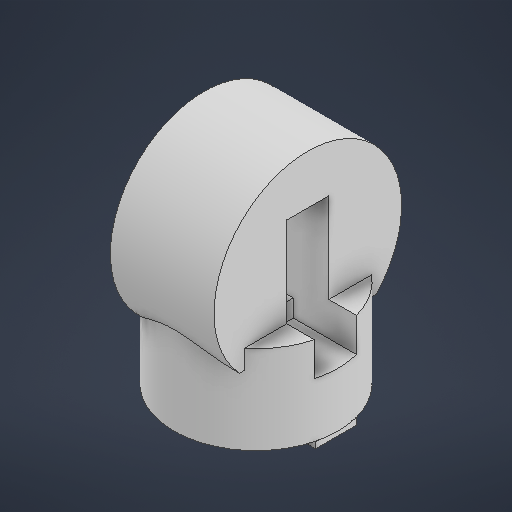
# Autodesk Inventor part: bottomPart
Saved by Autodesk Inventor 2026.2 (Build 302298000, 298)
## iProperties
Created: 2026-04-05
Part Number: bottomPart
Material: Generic
Document SubType Name: Modeling
Designer: Brian Wang
Density: 1 g/cm^3
Appearance: Default
Author: Brian Wang
Autodesk Inventor part; units mm, degrees
ref_plane "YZ Plane" through (0, 0, 0) normal (1, 0, 0) x (0, 1, 0)
ref_plane "XZ Plane" through (0, 0, 0) normal (0, 1, 0) x (-1, 0, 0)
ref_plane "XY Plane" through (0, 0, 0) normal (0, 0, 1) x (1, 0, 0)
sketch "Sketch1" plane through (0, 0, 0) normal (0, 1, 0) x (-1, 0, 0)
  line L0 (39, 10) -> (10, 10)
  line L1 (10, 10) -> (10, 30)
  line L2 (10, 30) -> (-10, 30)
  line L3 (-10, 30) -> (-10, 10)
  line L4 (-10, 10) -> (-39, 10)
  line L5 (-39, 10) -> (-39, -10)
  line L6 (-39, -10) -> (-10, -10)
  line L7 (-10, -10) -> (-10, -30)
  line L8 (-10, -30) -> (10, -30)
  line L9 (10, -30) -> (10, -10)
  line L10 (39, -10) -> (10, -10)
  line L11 (39, -10) -> (39, 10)
  circle A0 centre (25, 5) radius 1.375
  circle A1 centre (-25, 5) radius 1.375
  circle A2 centre (25, -5) radius 1.375
  circle A3 centre (-25, -5) radius 1.375
  point P0 (0, 0)
  dimension "d0" = 29
  dimension "d1" = 20
  dimension "d2" = 90
  dimension "d3" = 20
  dimension "d4" = 90
  dimension "d5" = 29
  dimension "d6" = 20
  dimension "d7" = 90
  dimension "d8" = 20
  dimension "d11" = 2.75
  dimension "d12" = 2.75
  dimension "d13" = 50
  dimension "d14" = 78
  dimension "d15" = 14
  dimension "d16" = 5
  dimension "d20" = 14
  dimension "d21" = 5
  dimension "d22" = 10
  dimension "d23" = 14
  dimension "d24" = 5
  dimension "d25" = 10
  dimension "d26" = 5
  constraints: 24 end point, 8 perpendicular, 8 point on line, 4 centre point, 1 horizontal
  measures "d0" distance of L0.start L0.end
  measures "d1" distance of L0.end L1.end
  measures "d2" angle of L0 L1
  measures "d3" distance of L1.end L2.end
  measures "d4" angle of L2 L1
  measures "d5" distance of L3.end L4.end
  measures "d6" distance of L4.end L5.end
  measures "d7" angle of L5 L4
  measures "d8" distance of L6.end L7.end
  measures "d11" diameter of A0
  measures "d12" diameter of A1
  measures "d13" distance of A1.centre A0.centre
  measures "d14" distance between parallel lines of L11 L5
  measures "d15" distance from line of L11 A0.centre
  measures "d16" distance from line of L0 A0.centre
  measures "d20" distance from line of L11 A2.centre
  measures "d21" distance from line of L10 A2.centre
  measures "d22" distance of A0.centre A2.centre
  measures "d23" distance from line of L5 A3.centre
  measures "d24" distance from line of L6 A3.centre
  measures "d25" distance of A3.centre A1.centre
  measures "d26" distance from line of L4 A1.centre
extrude "Extrusion1" add sketch "Sketch1" along normal blind 3
sketch "Sketch2" plane through (0, 3, 0) normal (0, 1, 0) x (1, 0, 0)
  circle A0 centre (0, 0) radius 40
  dimension "d27" = 80
  constraints: 1 centre point, 1 coincident
  measures "d27" diameter of A0
extrude "Extrusion2" add sketch "Sketch2" along normal blind 3
sketch "Sketch3" plane through (0, 6, 0) normal (0, 1, 0) x (1, 0, 0)
  circle A0 centre (0, 0) radius 40
  circle A1 centre (0, 0) radius 36.5
  dimension "d31" = 73
  constraints: 2 centre point, 2 coincident
  measures "d31" diameter of A1
extrude "Extrusion3" add sketch "Sketch3" along normal blind 40 contours A0 | A1
sketch "Sketch4" plane through (0, 46, 0) normal (0, 1, 0) x (1, 0, 0)
  line L0 (-19.25, 10.25) -> (19.25, 10.25)
  line L1 (19.25, 10.25) -> (19.25, -10.25)
  line L2 (19.25, -10.25) -> (-19.25, -10.25)
  line L3 (-19.25, -10.25) -> (-19.25, 10.25)
  point P0 (0, 0)
  dimension "d34" = 38.5
  dimension "d35" = 20.5
  dimension "d36" = 19.25
  dimension "d37" = 10.25
  constraints: 8 end point, 2 parallel, 1 horizontal, 1 perpendicular
  measures "d34" distance of L1.end L2.end
  measures "d35" distance of L0.end L1.end
  measures "d36" distance from line of L3 point (0, 0)
  measures "d37" distance from line of L0 point (0, 0)
extrude "Extrusion4" cut sketch "Sketch4" against normal blind 8
sketch "Sketch5" plane through (0, 38, 0) normal (0, 1, 0) x (1, 0, 0)
  line L0 (-19.25, 10.25) -> (19.25, 10.25) projected
  line L1 (19.25, -10.25) -> (-19.25, -10.25) projected
  line L2 (10.8, 10.25) -> (7.9, 10.25)
  line L3 (7.9, 10.25) -> (7.9, -10.25)
  line L4 (7.9, -10.25) -> (10.8, -10.25)
  line L5 (10.8, -10.25) -> (10.8, 10.25)
  line L6 (19.25, 10.25) -> (19.25, -10.25) projected
  line L7 (6.4, -10.25) -> (3.84, -10.25)
  line L8 (3.84, 10.25) -> (6.4, 10.25)
  point P0 (0, 0)
  dimension "d40" = 2.9
  dimension "d41" = 8.45
  constraints: 12 end point, 4 point on line, 3 parallel, 2 horizontal, 1 perpendicular
  measures "d40" distance of L4.end L3.end
  measures "d41" distance between parallel lines of L6 L5
extrude "Extrusion5" cut sketch "Sketch5" against normal blind 8.5 contours L0 L5 L1 L3
sketch "Sketch6" plane through (7.9, 38, 10.25) normal (1, 0, 0) x (0, 0, -1)
  line L0 (0, 0) -> (0, -8.5) projected
  line L1 (0, 0) -> (20.5, 0) projected
  line L2 (0, -8.5) -> (20.5, -8.5)
  line L3 (20.5, -8.5) -> (20.5, 0)
  line L4 (20.5, 0) -> (0, 0)
  line L5 (0, 0) -> (0, -8.5)
  point P0 (10.25, -38)
  constraints: 8 end point, 2 parallel, 1 horizontal, 1 perpendicular
extrude "Extrusion6" cut sketch "Sketch6" along normal blind 49
sketch "Sketch7" plane through (7.9, 38, 10.25) normal (1, 0, 0) x (0, 0, -1)
  circle A0 centre (5.25, -4.25) radius 1.35
  circle A1 centre (15.25, -4.25) radius 1.35
  line L0 (20.5, 0) -> (0, 0) projected
  line L1 (0, -8.5) -> (0, 0) projected
  point P0 (10.25, -38)
  dimension "d48" = 2.7
  dimension "d49" = 2.7
  dimension "d50" = 10
  dimension "d51" = 4.25
  dimension "d52" = 4.25
  dimension "d53" = 5.25
  constraints: 2 centre point
  measures "d48" diameter of A0
  measures "d49" diameter of A1
  measures "d50" distance of A0.centre A1.centre
  measures "d51" distance from line of L0 A0.centre
  measures "d52" distance from line of L0 A1.centre
  measures "d53" distance from line of L1 A0.centre
extrude "Extrusion7" cut sketch "Sketch7" against normal blind 7
sketch "Sketch8" plane through (0, 0, 0) normal (1, 0, 0) x (0, 1, 0)
  circle A0 centre (68, 0) radius 45.7097
  line L0 (29.5, 10.25) -> (29.5, -10.25) projected
  line L1 (29.5, -10.25) -> (77.6, -10.25)
  line L2 (77.6, -10.25) -> (77.6, 10.25)
  line L3 (77.6, 10.25) -> (29.5, 10.25)
  line L4 (29.5, 10.25) -> (29.5, -10.25)
  circle A1 centre (68, 0) radius 2.5
  point P0 (0, 0)
  dimension "d56" = 48.1
  dimension "d74" = 5
  constraints: 8 end point, 2 centre point, 2 parallel, 1 coincident, 1 horizontal, 1 perpendicular
  measures "d56" distance of L3.end L2.end
  measures "d74" diameter of A1
extrude "Extrusion8" add sketch "Sketch8" along normal mid plane 44.5 contours A0
sketch "Sketch9" plane through (0, 29.5, 0) normal (0, 1, 0) x (1, 0, 0)
  line L0 (22.25, -10.25) -> (22.25, 10.25) projected
  line L1 (7.9, -10.25) -> (7.9, 10.25) projected
  line L2 (22.25, 10.25) -> (7.9, 10.25)
  line L3 (7.9, 10.25) -> (7.9, -10.25)
  line L4 (7.9, -10.25) -> (22.25, -10.25)
  line L5 (22.25, -10.25) -> (22.25, 10.25)
  point P0 (0, 0)
  point P1 (22.25, -10.25)
  constraints: 8 end point, 2 parallel, 1 horizontal, 1 perpendicular
extrude "Extrusion9" cut sketch "Sketch9" along normal blind 56.1
sketch "Sketch10" plane through (0, 29.5, 0) normal (0, 1, 0) x (1, 0, 0)
  line L0 (22.25, 10.25) -> (22.25, -10.25) projected
  line L1 (22.25, -10.25) -> (93.4732, -10.25)
  line L2 (93.4732, -10.25) -> (93.4732, 10.25)
  line L3 (93.4732, 10.25) -> (22.25, 10.25)
  line L4 (22.25, 10.25) -> (22.25, -10.25)
  point P0 (0, 0)
  point P1 (22.25, 10.25)
  constraints: 8 end point, 2 parallel, 1 horizontal, 1 perpendicular
extrude "Extrusion10" cut sketch "Sketch10" along normal blind 32.85
sketch "Sketch11" plane through (7.9, 77.6, -10.25) normal (1, 0, 0) x (0, 0, -1)
  circle A0 centre (-15.25, -43.85) radius 1.35 projected
  circle A1 centre (-15.25, -43.85) radius 1.35
  circle A2 centre (-5.25, -43.85) radius 1.35 projected
  circle A3 centre (-5.25, -43.85) radius 1.35
  circle A4 centre (-15.25, 6.15) radius 1.35
  circle A5 centre (-5.25, 6.15) radius 1.35
  point P0 (-10.25, -77.6)
  dimension "d63" = 2.7
  dimension "d64" = 50
  dimension "d65" = 50
  constraints: 4 centre point, 2 coincident
  measures "d63" diameter of A4
  measures "d64" distance of A1.centre A4.centre
  measures "d65" distance of A3.centre A5.centre
sketch "Sketch12" plane through (22.25, 0, 0) normal (1, 0, 0) x (0, 0, -1)
  line L0 (-10.25, 85.6) -> (10.25, 85.6) projected
  line L1 (-10.25, 85.6) -> (10.25, 85.6)
  line L2 (10.25, 85.6) -> (10.25, 89.7782)
  line L3 (10.25, 89.7782) -> (-10.25, 89.7782)
  line L4 (-10.25, 89.7782) -> (-10.25, 85.6)
  point P0 (0, 0)
  constraints: 8 end point, 2 parallel, 1 horizontal, 1 perpendicular
sketch "Sketch13" plane through (7.9, 77.6, -10.25) normal (1, 0, 0) x (0, 0, -1)
  line L0 (0, 0) -> (-20.5, 0) projected
  line L1 (-20.5, -31.6) -> (-20.5, 8) projected
  line L2 (0, 0) -> (-20.5, 0)
  line L3 (-20.5, 0) -> (-20.5, 2.8423)
  line L4 (-20.5, 2.8423) -> (0, 2.8423)
  line L5 (0, 2.8423) -> (0, 0)
  point P0 (-10.25, -77.6)
  constraints: 8 end point, 2 parallel, 1 horizontal, 1 perpendicular, 1 point on line
extrude "Extrusion11" cut sketch "Sketch13" against normal blind 65.65
extrude "Extrusion12" cut sketch "Sketch12" against normal up to surface (14.35 mm away)
extrude "Extrusion13" cut sketch "Sketch11" against normal blind 7 contours A4 | A5
sketch "Sketch14" plane through (-22.25, 0, 0) normal (-1, 0, 0) x (0, 0, 1)
  line L0 (10.25, 80.4423) -> (-10.25, 80.4423) projected
  line L1 (33.2406, 46) -> (10.25, 46) projected
  line L2 (-10.25, 80.4423) -> (10.25, 80.4423)
  line L3 (10.25, 80.4423) -> (10.25, 46)
  line L4 (10.25, 46) -> (-10.25, 46)
  line L5 (-10.25, 46) -> (-10.25, 80.4423)
  point P0 (0, 0)
  constraints: 8 end point, 2 parallel, 1 horizontal, 1 perpendicular
extrude "Extrusion14" add sketch "Sketch14" against normal blind 3
sketch "Sketch15" plane through (-22.25, 0, 0) normal (-1, 0, 0) x (0, 0, 1)
  point P0 (0, 0)
sketch "Sketch16" plane through (-19.25, 38, 10.25) normal (1, 0, 0) x (0, 0, -1)
  circle A0 centre (10.25, 30.5) radius 3
  line L0 (0, 0) -> (20.5, 0) projected
  point P0 (10.25, -38)
  dimension "d75" = 6
  dimension "d76" = 30.5
  constraints: 1 centre point
  measures "d75" diameter of A0
  measures "d76" distance from line of L0 A0.centre
extrude "Extrusion15" cut sketch "Sketch16" against normal through all
sketch "Sketch17" plane through (-22.25, 0, 0) normal (-1, 0, 0) x (0, 0, 1)
  circle A0 centre (0, 68.5) radius 3 projected
  circle A1 centre (0, 68.5) radius 3
  arc A2 (33.2406, 36.6242) -> (-33.2406, 36.6242) centre (0, 68) ccw projected
  line L0 (-33.2406, 46) -> (-33.2406, 36.6242) projected
  arc A3 (0, 113.7097) -> (-33.2406, 36.6242) centre (0, 68) ccw
  arc A4 (33.2406, 36.6242) -> (0, 113.7097) centre (0, 68) ccw
  line L1 (33.2406, 46) -> (-33.2406, 46) projected
  line L2 (-33.2406, 46) -> (33.2406, 46)
  line L3 (33.2406, 46) -> (33.2406, 36.6242)
  point P0 (0, 0)
  dimension "d79" = 6
  constraints: 5 point on circle, 4 end point, 3 centre point, 3 concentric, 1 collinear, 1 perpendicular
  measures "d79" diameter of A1
extrude "Extrusion16" add sketch "Sketch17" along normal blind 3
sketch "Sketch18" plane through (22.25, 0, 0) normal (1, 0, 0) x (0, 0, -1)
  line L0 (-33.2406, 46) -> (-33.2406, 36.6242) projected
  line L1 (33.2406, 46) -> (33.2406, 36.6242) projected
  line L2 (-33.2406, 36.6242) -> (-33.2406, 46)
  line L3 (-10.25, 46) -> (-33.2406, 46) projected
  line L4 (-10.25, 89.7782) -> (10.25, 89.7782) projected
  line L5 (-10.25, 46) -> (-10.25, 89.7782)
  line L6 (-10.25, 89.7782) -> (10.25, 89.7782)
  line L7 (10.25, 89.7782) -> (10.25, 46)
  line L8 (10.25, 46) -> (33.2406, 46)
  arc A0 (33.2406, 36.6242) -> (-33.2406, 36.6242) centre (0, 68) ccw projected
  arc A1 (0, 113.7097) -> (-33.2406, 36.6242) centre (0, 68) ccw
  arc A2 (33.2406, 36.6242) -> (0, 113.7097) centre (0, 68) ccw
  point P0 (0, 0)
  constraints: 10 end point, 5 point on circle, 2 centre point, 2 collinear, 2 perpendicular, 1 concentric, 1 vertical
extrude "Extrusion17" add sketch "Sketch18" along normal blind 3
sketch "Sketch20" plane through (22.25, 36.6242, -33.2406) normal (0, 0, 1) x (1, 0, 0)
  line L0 (3, 0) -> (3, 77.0854) projected
  line L1 (3, 9.3758) -> (0, 9.3758) projected
  line L2 (3, 0) -> (0, 0)
  line L3 (0, 0) -> (0, 9.3758)
  line L4 (0, 9.3758) -> (3, 9.3758)
  line L5 (3, 9.3758) -> (3, 0)
  point P0 (-22.25, -36.6242)
  constraints: 8 end point, 2 parallel, 1 horizontal, 1 perpendicular
extrude "Extrusion18" add sketch "Sketch20" along normal blind 3
sketch "Sketch21" plane through (25.25, 46, 33.2406) normal (0, 0, -1) x (-1, 0, 0)
  line L0 (3, -9.3758) -> (0, -9.3758) projected
  line L1 (0, -9.3758) -> (6.3814, -9.3758)
  line L2 (6.3814, -9.3758) -> (6.3814, 0.5488)
  line L3 (6.3814, 0.5488) -> (0, 0.5488)
  line L4 (0, 0.5488) -> (0, -9.3758)
  point P0 (25.25, -46)
  constraints: 8 end point, 2 parallel, 1 horizontal, 1 perpendicular
extrude "Extrusion19" add sketch "Sketch21" along normal blind 3.75
sketch "Sketch22" plane through (-25.25, 46, -33.2406) normal (0, 0, 1) x (1, 0, 0)
  line L0 (3, -9.3758) -> (0, -9.3758) projected
  line L1 (3, 0) -> (0, 0) projected
  line L2 (0, -9.3758) -> (3, -9.3758)
  line L3 (3, -9.3758) -> (3, 0)
  line L4 (3, 0) -> (0, 0)
  line L5 (0, 0) -> (0, -9.3758)
  point P0 (25.25, -46)
  constraints: 8 end point, 2 parallel, 1 horizontal, 1 perpendicular
extrude "Extrusion20" add sketch "Sketch22" along normal blind 3.75
sketch "Sketch23" plane through (-22.25, 36.6242, 33.2406) normal (0, 0, -1) x (-1, 0, 0)
  line L0 (0, 0) -> (3, 0) projected
  line L1 (3, 9.3758) -> (0, 9.3758)
  line L2 (0, 9.3758) -> (0, 0)
  line L3 (0, 0) -> (3, 0)
  line L4 (3, 0) -> (3, 9.3758)
  point P0 (-22.25, -36.6242)
  constraints: 8 end point, 2 parallel, 1 horizontal, 1 perpendicular
extrude "Extrusion21" add sketch "Sketch23" along normal blind 3.75
body "Solid1"
